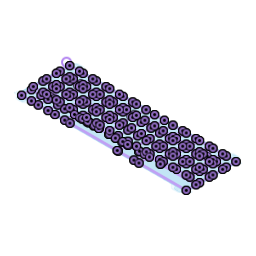
All_Plates (Autodesk Fusion 360 design; units mm, degrees)
Autodesk Fusion 360 part; units mm, degrees
(part 1 of 6)
sketch "campsite" plane through (0, 0, 0) normal (0, 1, 0) x (1, 0, 0)
  arc A0 (-6.7013, -67.15) -> (-8.4334, -66.15) centre (-8.4334, -68.15) ccw
  arc A1 (-9, 8.5) -> (-8.5, 9) centre (-8.5, 8.5) cw
  line L0 (-4.3919, 14) -> (3.6799, 14)
  arc A2 (-8.5, -66.15) -> (-9, -65.65) centre (-8.5, -65.65) cw
  line L1 (-8.5, 9) -> (-8.4334, 9)
  arc A3 (216.1161, 9) -> (217.8482, 10) centre (216.1161, 11) ccw
  line L2 (-6.7013, 10) -> (-4.3919, 14)
  line L3 (7.7214, 9) -> (216.1161, 9)
  arc A4 (-8.4334, 9) -> (-6.7013, 10) centre (-8.4334, 11) ccw
  arc A5 (232.8375, -65.65) -> (232.3375, -66.15) centre (232.3375, -65.65) cw
  line L4 (3.6799, 14) -> (5.9893, 10)
  line L5 (217.8482, 10) -> (220.1576, 14)
  line L6 (232.3375, -66.15) -> (232.2709, -66.15)
  line L7 (232.2709, 9) -> (232.3375, 9)
  arc A6 (217.8482, -67.15) -> (216.1161, -66.15) centre (216.1161, -68.15) ccw
  line L8 (-8.4334, -66.15) -> (-8.5, -66.15)
  arc A7 (7.7214, -66.15) -> (5.9893, -67.15) centre (7.7214, -68.15) ccw
  line L9 (220.1576, -71.15) -> (217.8482, -67.15)
  line L10 (-4.3919, -71.15) -> (-6.7013, -67.15)
  line L11 (-9, -65.65) -> (-9, 8.5)
  arc A8 (5.9893, 10) -> (7.7214, 9) centre (7.7214, 11) ccw
  arc A9 (232.2709, -66.15) -> (230.5388, -67.15) centre (232.2709, -68.15) ccw
  line L12 (232.8375, 8.5) -> (232.8375, -65.65)
  line L13 (228.2294, 14) -> (230.5388, 10)
  arc A10 (232.3375, 9) -> (232.8375, 8.5) centre (232.3375, 8.5) cw
  line L14 (5.9893, -67.15) -> (3.6799, -71.15)
  line L15 (216.1161, -66.15) -> (7.7214, -66.15)
  line L16 (228.2294, -71.15) -> (220.1576, -71.15)
  arc A11 (230.5388, 10) -> (232.2709, 9) centre (232.2709, 11) ccw
  line L17 (230.5388, -67.15) -> (228.2294, -71.15)
  line L18 (3.6799, -71.15) -> (-4.3919, -71.15)
  line L19 (220.1576, 14) -> (228.2294, 14)
sketch "coriander" plane through (0, 0, 0) normal (0, 1, 0) x (1, 0, 0)
  arc A0 (13.2901, -66.675) -> (10.6915, -67.7514) centre (13.2901, -70.35) ccw
  arc A1 (213.146, -67.7514) -> (210.5474, -66.675) centre (210.5474, -70.35) ccw
  line L0 (-9.525, -65.8599) -> (-9.525, 8.7099)
  arc A2 (226.5474, 15.525) -> (228.4389, 14.7415) centre (226.5474, 12.85) cw
  line L1 (228.4389, 14.7415) -> (232.579, 10.6014)
  line L2 (233.3625, 8.7099) -> (233.3625, -65.8599)
  arc A3 (232.579, 10.6014) -> (233.3625, 8.7099) centre (230.6875, 8.7099) cw
  line L3 (217.2861, -71.8915) -> (213.146, -67.7514)
  line L4 (213.114, 10.5694) -> (217.2861, 14.7415)
  line L5 (6.5514, 14.7415) -> (10.6915, 10.6014)
  arc A4 (-8.7415, -67.7514) -> (-9.525, -65.8599) centre (-6.85, -65.8599) cw
  arc A5 (210.5474, 9.525) -> (213.1139, 10.5697) centre (210.5474, 13.2) ccw
  arc A6 (10.6915, 10.6014) -> (13.2901, 9.525) centre (13.2901, 13.2) ccw
  arc A7 (-2.7099, -72.675) -> (-4.6014, -71.8915) centre (-2.7099, -70) cw
  arc A8 (6.5514, -71.8915) -> (4.6599, -72.675) centre (4.6599, -70) cw
  arc A9 (217.2861, 14.7415) -> (219.1776, 15.525) centre (219.1776, 12.85) cw
  line L6 (219.1776, 15.525) -> (226.5474, 15.525)
  arc A10 (228.4389, -71.8915) -> (226.5474, -72.675) centre (226.5474, -70) cw
  line L7 (10.6915, -67.7514) -> (6.5514, -71.8915)
  circle A11 centre (0.9751, -69.925) radius 1.25
  line L8 (-8.7415, 10.6014) -> (-4.6014, 14.7415)
  line L9 (232.579, -67.7514) -> (228.4389, -71.8915)
  arc A12 (-4.6014, 14.7415) -> (-2.7099, 15.525) centre (-2.7099, 12.85) cw
  arc A13 (233.3625, -65.8599) -> (232.579, -67.7514) centre (230.6875, -65.8599) cw
  arc A14 (219.1776, -72.675) -> (217.2861, -71.8915) centre (219.1776, -70) cw
  circle A15 centre (222.8626, -69.925) radius 1.25
  line L10 (-4.6014, -71.8915) -> (-8.7415, -67.7514)
  arc A16 (-9.525, 8.7099) -> (-8.7415, 10.6014) centre (-6.85, 8.7099) cw
  line L11 (-2.7099, 15.525) -> (4.6599, 15.525)
  line L12 (4.6599, -72.675) -> (-2.7099, -72.675)
  line L13 (226.5474, -72.675) -> (219.1776, -72.675)
  circle A17 centre (0.9749, 12.775) radius 1.25
  arc A18 (4.6599, 15.525) -> (6.5514, 14.7415) centre (4.6599, 12.85) cw
  line L14 (13.2901, 9.525) -> (210.5474, 9.525)
  arc A19 (213.1139, 10.5697) -> (213.114, 10.5694) centre (210.5375, 9.85) cw
  line L15 (210.5474, -66.675) -> (13.2901, -66.675)
  circle A20 centre (222.8624, 12.775) radius 1.25
sketch "hull" plane through (130.0399, 0, -35.1845) normal (0, 1, 0) x (1, 0, 0)
  arc A0 (107.0801, -27.1082) -> (107.0801, -29.5607) centre (107.3226, -28.3345) ccw
  arc A1 (104.8226, -31.0095) -> (103.3226, -32.5095) centre (104.8226, -32.5095) ccw
  line L0 (103.3226, -95.0095) -> (103.3226, -32.5095)
  line L1 (104.8226, -31.0095) -> (105.6476, -31.0095)
  arc A2 (105.6476, -31.0095) -> (107.2901, -30.4459) centre (105.6476, -28.3345) ccw
  arc A3 (107.2901, -30.4459) -> (107.0801, -29.5607) centre (106.9831, -30.0512) ccw
  arc A4 (-141.8899, -25.6595) -> (-143.5323, -26.2231) centre (-141.8899, -28.3345) ccw
  arc A5 (-143.3224, -29.5607) -> (-143.3224, -27.1082) centre (-143.5649, -28.3345) ccw
  arc A6 (-143.5323, -30.4459) -> (-141.8899, -31.0095) centre (-141.8899, -28.3345) ccw
  arc A7 (107.2901, -26.2231) -> (105.6476, -25.6595) centre (105.6476, -28.3345) ccw
  arc A8 (-139.5649, -32.5095) -> (-141.0649, -31.0095) centre (-141.0649, -32.5095) ccw
  arc A9 (107.0801, -27.1082) -> (107.2901, -26.2231) centre (106.9831, -26.6177) ccw
  line L2 (-139.5649, -32.5095) -> (-139.5649, -95.0095)
  line L3 (-141.0649, -96.5095) -> (-141.8899, -96.5095)
  arc A10 (-143.5323, -26.2231) -> (-143.3224, -27.1082) centre (-143.2253, -26.6177) ccw
  arc A11 (-143.3224, -29.5607) -> (-143.5323, -30.4459) centre (-143.2253, -30.0512) ccw
  line L4 (105.6476, -25.6595) -> (-141.8899, -25.6595)
  arc A12 (-141.0649, -96.5095) -> (-139.5649, -95.0095) centre (-141.0649, -95.0095) ccw
  line L5 (-141.8899, -31.0095) -> (-141.0649, -31.0095)
  arc A13 (107.2901, -101.2959) -> (107.0801, -100.4107) centre (106.9831, -100.9012) ccw
  arc A14 (107.2901, -97.0731) -> (105.6476, -96.5095) centre (105.6476, -99.1845) ccw
  arc A15 (-143.3224, -100.4107) -> (-143.3224, -97.9582) centre (-143.5649, -99.1845) ccw
  arc A16 (-141.8899, -96.5095) -> (-143.5323, -97.0731) centre (-141.8899, -99.1845) ccw
  arc A17 (-143.5323, -97.0731) -> (-143.3224, -97.9582) centre (-143.2253, -97.4677) ccw
  line L6 (-141.8899, -101.8595) -> (105.6476, -101.8595)
  arc A18 (103.3226, -95.0095) -> (104.8226, -96.5095) centre (104.8226, -95.0095) ccw
  arc A19 (-143.3224, -100.4107) -> (-143.5323, -101.2959) centre (-143.2253, -100.9012) ccw
  arc A20 (105.6476, -101.8595) -> (107.2901, -101.2959) centre (105.6476, -99.1845) ccw
  arc A21 (107.0801, -97.9582) -> (107.2901, -97.0731) centre (106.9831, -97.4677) ccw
  line L7 (105.6476, -96.5095) -> (104.8226, -96.5095)
  arc A22 (107.0801, -97.9582) -> (107.0801, -100.4107) centre (107.3226, -99.1845) ccw
  arc A23 (-143.5323, -101.2959) -> (-141.8899, -101.8595) centre (-141.8899, -99.1845) ccw
  point P0 (-130.0399, -35.1845)
sketch "tray" plane through (-50, 0, 0) normal (0, 1, 0) x (1, 0, 0)
  line L0 (43.225, 9.5245) -> (280.6123, 9.5245)
  line L1 (280.6123, -66.6754) -> (43.225, -66.6754)
  line L2 (283.6123, 6.5245) -> (283.6123, -63.6754)
  arc A0 (280.6123, 9.5245) -> (283.6123, 6.5245) centre (280.6123, 6.5245) cw
  arc A1 (283.6123, -63.6754) -> (280.6123, -66.6754) centre (280.6123, -63.6754) cw
  arc A2 (43.225, -66.6754) -> (40.225, -63.6754) centre (43.225, -63.6754) cw
  circle A3 centre (70.325, -44.2754) radius 2.75
  line L3 (40.225, -63.6754) -> (40.225, 6.5245)
  circle A4 centre (117.225, -55.8254) radius 2.75
  arc A5 (40.225, 6.5245) -> (43.225, 9.5245) centre (43.225, 6.5245) cw
  circle A6 centre (222.8123, -56.0254) radius 2.75
  circle A7 centre (251.1123, -7.2255) radius 2.75
  circle A8 centre (71.875, -9.5255) radius 2.75
  circle A9 centre (148.075, -9.5255) radius 2.75
  circle A10 centre (178.5623, -28.6255) radius 2.75
  point P0 (50, 0)
extrude "Extrude1" add sketch "campsite" along normal blind 10 makes body 1
extrude "Extrude2" add sketch "coriander" along normal blind 10 separate body contours A0 A1 L0 A2 L1 L2 A3 L3 L4 L5 A4 A6 A7 A8 A9 L6 A10 L7 L8 L9 A12 A13 A14 L10 A16 L11 L12 L13 A18 L14 A19 L15 | A5 L14 A19 picked at (210.945, 8.7857) makes body 2
extrude "Extrude3" add sketch "hull" along normal blind 10 separate body makes body 3
extrude "Extrude4" add sketch "tray" along normal blind 10 separate body makes body 4
copy_body "CopyPasteBodies1" bodies 2 makes body 5
move_body "Move1" bodies 5 to x (1, 0, 0) y (0, 1, 0) z (0, 0, 1) at (0, 0, 0)
combine "Combine1" operation intersect target body 5 tool bodies 1 keep tools
copy_body "CopyPasteBodies3" bodies 3 makes body 6
move_body "Move3" bodies 6 to x (1, 0, 0) y (0, 1, 0) z (0, 0, 1) at (0, 0, 0)
extrude "Extrude5" cut sketch "tray" along normal blind 10 contours A3 | A4 | A6 | A7 | A8 | A9 | A10 bodies 6
sketch "campiander" plane through (0, 0, 0) normal (0, 1, 0) x (1, 0, 0)
  line L0 (217.8482, 10) -> (220.1576, 14)
  arc A0 (-6.7013, -67.15) -> (-8.4334, -66.15) centre (-8.4334, -68.15) ccw
  line L1 (222.6139, -71.15) -> (220.1576, -71.15)
  line L2 (220.1576, -71.15) -> (217.8482, -67.15)
  arc A1 (222.6136, 14) -> (223.1111, 14) centre (222.8624, 12.775) ccw
  arc A2 (-8.5, -66.15) -> (-9, -65.65) centre (-8.5, -65.65) cw
  arc A3 (230.5388, 10) -> (232.2709, 9) centre (232.2709, 11) ccw
  arc A4 (-8.4334, 9) -> (-6.7013, 10) centre (-8.4334, 11) ccw
  arc A5 (217.8482, -67.15) -> (216.1161, -66.15) centre (216.1161, -68.15) ccw
  line L3 (232.3375, -66.15) -> (232.2709, -66.15)
  line L4 (-4.3919, 14) -> (0.7261, 14)
  line L5 (-9, -65.65) -> (-9, 8.5)
  line L6 (5.9893, -67.15) -> (3.6799, -71.15)
  line L7 (-8.4334, -66.15) -> (-8.5, -66.15)
  line L8 (-8.5, 9) -> (-8.4334, 9)
  line L9 (7.7214, 9) -> (216.1161, 9)
  arc A6 (232.2709, -66.15) -> (230.5388, -67.15) centre (232.2709, -68.15) ccw
  arc A7 (0.7261, 14) -> (1.2236, 14) centre (0.9749, 12.775) ccw
  arc A8 (1.2239, -71.15) -> (0.7264, -71.15) centre (0.9751, -69.925) ccw
  line L10 (223.1111, 14) -> (228.2294, 14)
  line L11 (228.2294, 14) -> (230.5388, 10)
  arc A9 (232.3375, 9) -> (232.8375, 8.5) centre (232.3375, 8.5) cw
  line L12 (232.8375, 8.5) -> (232.8375, -65.65)
  arc A10 (-9, 8.5) -> (-8.5, 9) centre (-8.5, 8.5) cw
  line L13 (-6.7013, 10) -> (-4.3919, 14)
  line L14 (0.7264, -71.15) -> (-4.3919, -71.15)
  line L15 (232.2709, 9) -> (232.3375, 9)
  line L16 (1.2236, 14) -> (3.6799, 14)
  line L17 (3.6799, 14) -> (5.9893, 10)
  arc A11 (216.1161, 9) -> (217.8482, 10) centre (216.1161, 11) ccw
  line L18 (220.1576, 14) -> (222.6136, 14)
  line L19 (228.2294, -71.15) -> (223.1114, -71.15)
  line L20 (230.5388, -67.15) -> (228.2294, -71.15)
  line L21 (3.6799, -71.15) -> (1.2239, -71.15)
  line L22 (216.1161, -66.15) -> (7.7214, -66.15)
  arc A12 (5.9893, 10) -> (7.7214, 9) centre (7.7214, 11) ccw
  arc A13 (232.8375, -65.65) -> (232.3375, -66.15) centre (232.3375, -65.65) cw
  arc A14 (7.7214, -66.15) -> (5.9893, -67.15) centre (7.7214, -68.15) ccw
  arc A15 (223.1114, -71.15) -> (222.6139, -71.15) centre (222.8626, -69.925) ccw
  line L23 (-4.3919, -71.15) -> (-6.7013, -67.15)
sketch "minisub" plane through (22.36, 0, 75.2938) normal (0, 1, 0) x (1, 0, 0)
  line L0 (52.5458, 11.1438) -> (52.5458, 26.1438)
  line L1 (115.6088, 25.1438) -> (101.6088, 25.1438)
  line L2 (208.4775, 11.1438) -> (208.4775, 25.1438)
  line L3 (140.8213, 26.1438) -> (140.8213, 25.1438)
  line L4 (45.5458, 26.1438) -> (40.8213, 26.1438)
  line L5 (76.4218, 26.1438) -> (69.4218, 26.1438)
  line L6 (100.1708, 26.1438) -> (93.1708, 26.1438)
  line L7 (52.5458, 26.1438) -> (47.8213, 26.1438)
  line L8 (100.1708, 11.1438) -> (101.6088, 11.1438)
  line L9 (147.8213, 26.1438) -> (140.8213, 26.1438)
  line L10 (147.8213, 25.1438) -> (147.8213, 26.1438)
  line L11 (67.9838, 25.1438) -> (53.9838, 25.1438)
  line L12 (148.9463, 11.1438) -> (148.9463, 25.1438)
  line L13 (47.8213, 11.1438) -> (52.5458, 11.1438)
  line L14 (101.6088, 25.1438) -> (100.1708, 25.1438)
  line L15 (208.4775, 25.1438) -> (194.4775, 25.1438)
  line L16 (47.8213, 26.1438) -> (45.5458, 26.1438)
  line L17 (53.9838, 11.1438) -> (67.9838, 11.1438)
  line L18 (115.6088, 11.1438) -> (115.6088, 25.1438)
  line L19 (147.8213, 11.1438) -> (148.9463, 11.1438)
  line L20 (124.0468, 11.1438) -> (124.0468, 26.1438)
  line L21 (175.4275, 11.1438) -> (189.4275, 11.1438)
  line L22 (69.4218, 11.1438) -> (76.4218, 11.1438)
  line L23 (194.4775, 25.1438) -> (194.4775, 11.1438)
  line L24 (189.4275, 11.1438) -> (189.4275, 25.1438)
  line L25 (93.1708, 25.1438) -> (87.3213, 25.1438)
  line L26 (189.4275, 25.1438) -> (175.4275, 25.1438)
  line L27 (69.4218, 26.1438) -> (69.4218, 11.1438)
  line L28 (170.3775, 25.1438) -> (156.3775, 25.1438)
  line L29 (93.1708, 26.1438) -> (93.1708, 25.1438)
  line L30 (156.3775, 11.1438) -> (170.3775, 11.1438)
  line L31 (93.1708, 11.1438) -> (100.1708, 11.1438)
  line L32 (53.9838, 25.1438) -> (53.9838, 11.1438)
  line L33 (45.5458, 11.1438) -> (47.8213, 11.1438)
  line L34 (124.0468, 26.1438) -> (117.0468, 26.1438)
  line L35 (140.8213, 25.1438) -> (134.9463, 25.1438)
  line L36 (175.4275, 25.1438) -> (175.4275, 11.1438)
  line L37 (117.0468, 11.1438) -> (124.0468, 11.1438)
  line L38 (76.4218, 11.1438) -> (76.4218, 26.1438)
  line L39 (140.8213, 11.1438) -> (147.8213, 11.1438)
  line L40 (134.9463, 11.1438) -> (140.8213, 11.1438)
  line L41 (65.89, 82.2938) -> (65.89, 68.2938)
  line L42 (142.09, 82.2938) -> (142.09, 68.2938)
  line L43 (175.14, 82.2938) -> (161.14, 82.2938)
  line L44 (46.84, 68.2938) -> (60.84, 68.2938)
  line L45 (84.94, 68.2938) -> (98.94, 68.2938)
  line L46 (8.74, 82.2938) -> (8.74, 68.2938)
  line L47 (117.99, 82.2938) -> (103.99, 82.2938)
  line L48 (98.94, 68.2938) -> (98.94, 82.2938)
  line L49 (123.04, 82.2938) -> (123.04, 68.2938)
  line L50 (41.79, 82.2938) -> (27.79, 82.2938)
  line L51 (79.89, 68.2938) -> (79.89, 82.2938)
  line L52 (27.79, 68.2938) -> (41.79, 68.2938)
  line L53 (161.14, 68.2938) -> (175.14, 68.2938)
  line L54 (13.5025, 49.2438) -> (27.5025, 49.2438)
  line L55 (175.14, 68.2938) -> (175.14, 82.2938)
  line L56 (46.84, 82.2938) -> (46.84, 68.2938)
  line L57 (65.89, 68.2938) -> (79.89, 68.2938)
  line L58 (103.99, 68.2938) -> (117.99, 68.2938)
  line L59 (41.79, 68.2938) -> (41.79, 82.2938)
  line L60 (98.94, 82.2938) -> (84.94, 82.2938)
  line L61 (117.99, 68.2938) -> (117.99, 82.2938)
  line L62 (142.09, 68.2938) -> (156.09, 68.2938)
  line L63 (60.84, 68.2938) -> (60.84, 82.2938)
  line L64 (22.74, 82.2938) -> (8.74, 82.2938)
  line L65 (156.09, 68.2938) -> (156.09, 82.2938)
  line L66 (187.3338, 68.2938) -> (201.3338, 68.2938)
  line L67 (3.69, 82.2938) -> (-10.31, 82.2938)
  line L68 (187.3338, 82.2938) -> (187.3338, 68.2938)
  line L69 (84.94, 82.2938) -> (84.94, 68.2938)
  line L70 (137.04, 82.2938) -> (123.04, 82.2938)
  line L71 (22.74, 68.2938) -> (22.74, 82.2938)
  line L72 (137.04, 68.2938) -> (137.04, 82.2938)
  line L73 (103.99, 82.2938) -> (103.99, 68.2938)
  line L74 (-10.31, 82.2938) -> (-10.31, 68.2938)
  line L75 (60.84, 82.2938) -> (46.84, 82.2938)
  line L76 (-26.9787, 49.2438) -> (-12.9787, 49.2438)
  line L77 (8.74, 68.2938) -> (22.74, 68.2938)
  line L78 (201.3338, 82.2938) -> (187.3338, 82.2938)
  line L79 (123.04, 68.2938) -> (137.04, 68.2938)
  line L80 (156.09, 82.2938) -> (142.09, 82.2938)
  line L81 (201.3338, 68.2938) -> (201.3338, 82.2938)
  line L82 (-12.9787, 63.2438) -> (-26.9787, 63.2438)
  line L83 (-12.9787, 49.2438) -> (-12.9787, 63.2438)
  line L84 (79.89, 82.2938) -> (65.89, 82.2938)
  line L85 (161.14, 82.2938) -> (161.14, 68.2938)
  line L86 (3.69, 68.2938) -> (3.69, 82.2938)
  line L87 (-26.9787, 63.2438) -> (-26.9787, 49.2438)
  line L88 (27.79, 82.2938) -> (27.79, 68.2938)
  line L89 (-5.5475, 49.2438) -> (8.4525, 49.2438)
  line L90 (8.4525, 49.2438) -> (8.4525, 63.2438)
  line L91 (-5.5475, 63.2438) -> (-5.5475, 49.2438)
  line L92 (8.4525, 63.2438) -> (-5.5475, 63.2438)
  line L93 (27.5025, 63.2438) -> (13.5025, 63.2438)
  line L94 (13.5025, 63.2438) -> (13.5025, 49.2438)
  line L95 (27.5025, 49.2438) -> (27.5025, 63.2438)
  line L96 (46.5525, 63.2438) -> (32.5525, 63.2438)
  line L97 (32.5525, 49.2438) -> (46.5525, 49.2438)
  line L98 (146.8525, 49.2438) -> (160.8525, 49.2438)
  line L99 (70.6525, 49.2438) -> (84.6525, 49.2438)
  line L100 (46.5525, 49.2438) -> (46.5525, 63.2438)
  line L101 (32.5525, 63.2438) -> (32.5525, 49.2438)
  line L102 (179.9025, 49.2438) -> (179.9025, 63.2438)
  line L103 (127.8025, 49.2438) -> (141.8025, 49.2438)
  line L104 (165.9025, 49.2438) -> (179.9025, 49.2438)
  line L105 (65.6025, 49.2438) -> (65.6025, 63.2438)
  line L106 (70.6525, 63.2438) -> (70.6525, 49.2438)
  line L107 (122.7525, 63.2438) -> (108.7525, 63.2438)
  line L108 (127.8025, 63.2438) -> (127.8025, 49.2438)
  line L109 (103.7025, 49.2438) -> (103.7025, 63.2438)
  line L110 (165.9025, 63.2438) -> (165.9025, 49.2438)
  line L111 (189.715, 49.2438) -> (203.715, 49.2438)
  line L112 (146.8525, 63.2438) -> (146.8525, 49.2438)
  line L113 (51.6025, 63.2438) -> (51.6025, 49.2438)
  line L114 (160.8525, 63.2438) -> (146.8525, 63.2438)
  line L115 (65.6025, 63.2438) -> (51.6025, 63.2438)
  line L116 (141.8025, 63.2438) -> (127.8025, 63.2438)
  line L117 (160.8525, 49.2438) -> (160.8525, 63.2438)
  line L118 (84.6525, 63.2438) -> (70.6525, 63.2438)
  line L119 (141.8025, 49.2438) -> (141.8025, 63.2438)
  line L120 (89.7025, 63.2438) -> (89.7025, 49.2438)
  line L121 (84.6525, 49.2438) -> (84.6525, 63.2438)
  line L122 (170.3775, 44.1938) -> (156.3775, 44.1938)
  line L123 (170.3775, 30.1938) -> (170.3775, 44.1938)
  line L124 (189.4275, 44.1938) -> (175.4275, 44.1938)
  line L125 (103.7025, 63.2438) -> (89.7025, 63.2438)
  line L126 (156.3775, 30.1938) -> (170.3775, 30.1938)
  line L127 (175.4275, 44.1938) -> (175.4275, 30.1938)
  line L128 (208.4775, 44.1938) -> (194.4775, 44.1938)
  line L129 (17.9775, 30.1938) -> (17.9775, 44.1938)
  line L130 (108.7525, 49.2438) -> (122.7525, 49.2438)
  line L131 (56.0775, 44.1938) -> (42.0775, 44.1938)
  line L132 (-8.2162, 30.1938) -> (-8.2162, 44.1938)
  line L133 (108.7525, 63.2438) -> (108.7525, 49.2438)
  line L134 (51.6025, 49.2438) -> (65.6025, 49.2438)
  line L135 (89.7025, 49.2438) -> (103.7025, 49.2438)
  line L136 (122.7525, 49.2438) -> (122.7525, 63.2438)
  line L137 (179.9025, 63.2438) -> (165.9025, 63.2438)
  line L138 (208.4775, 30.1938) -> (208.4775, 44.1938)
  line L139 (-12.9787, 11.1438) -> (-12.9787, 25.1438)
  line L140 (8.4525, 25.1438) -> (-5.5475, 25.1438)
  line L141 (80.1775, 30.1938) -> (94.1775, 30.1938)
  line L142 (99.2275, 44.1938) -> (99.2275, 30.1938)
  line L143 (175.4275, 30.1938) -> (189.4275, 30.1938)
  line L144 (8.4525, 11.1438) -> (8.4525, 25.1438)
  line L145 (-22.2162, 44.1938) -> (-22.2162, 30.1938)
  line L146 (137.3275, 44.1938) -> (137.3275, 30.1938)
  line L147 (-26.9787, 11.1438) -> (-12.9787, 11.1438)
  line L148 (-29.36, 68.2938) -> (-15.36, 68.2938)
  line L149 (-29.36, 82.2938) -> (-29.36, 68.2938)
  line L150 (-10.31, 68.2938) -> (3.69, 68.2938)
  line L151 (-15.36, 82.2938) -> (-29.36, 82.2938)
  line L152 (-15.36, 68.2938) -> (-15.36, 82.2938)
  line L153 (151.3275, 30.1938) -> (151.3275, 44.1938)
  line L154 (-8.2162, 44.1938) -> (-22.2162, 44.1938)
  line L155 (148.9463, 25.1438) -> (147.8213, 25.1438)
  line L156 (75.1275, 44.1938) -> (61.1275, 44.1938)
  line L157 (40.8213, 26.1438) -> (40.8213, 11.1438)
  line L158 (67.9838, 11.1438) -> (67.9838, 25.1438)
  line L159 (156.3775, 25.1438) -> (156.3775, 11.1438)
  line L160 (117.0468, 26.1438) -> (117.0468, 11.1438)
  line L161 (87.3213, 25.1438) -> (87.3213, 11.1438)
  line L162 (134.9463, 25.1438) -> (134.9463, 11.1438)
  line L163 (170.3775, 11.1438) -> (170.3775, 25.1438)
  line L164 (42.0775, 30.1938) -> (56.0775, 30.1938)
  line L165 (118.2775, 44.1938) -> (118.2775, 30.1938)
  line L166 (113.2275, 30.1938) -> (113.2275, 44.1938)
  line L167 (100.1708, 25.1438) -> (100.1708, 26.1438)
  line L168 (40.8213, 11.1438) -> (45.5458, 11.1438)
  line L169 (194.4775, 11.1438) -> (208.4775, 11.1438)
  line L170 (101.6088, 11.1438) -> (115.6088, 11.1438)
  line L171 (87.3213, 11.1438) -> (93.1708, 11.1438)
  line L172 (15.8838, 25.1438) -> (15.8838, 11.1438)
  line L173 (94.1775, 44.1938) -> (80.1775, 44.1938)
  line L174 (29.8838, 11.1438) -> (29.8838, 25.1438)
  line L175 (15.8838, 11.1438) -> (29.8838, 11.1438)
  line L176 (-5.5475, 25.1438) -> (-5.5475, 11.1438)
  line L177 (203.715, 63.2438) -> (189.715, 63.2438)
  line L178 (189.4275, 30.1938) -> (189.4275, 44.1938)
  line L179 (156.3775, 44.1938) -> (156.3775, 30.1938)
  line L180 (194.4775, 30.1938) -> (208.4775, 30.1938)
  line L181 (29.8838, 25.1438) -> (15.8838, 25.1438)
  line L182 (194.4775, 44.1938) -> (194.4775, 30.1938)
  line L183 (-5.5475, 11.1438) -> (8.4525, 11.1438)
  line L184 (-12.9787, 25.1438) -> (-26.9787, 25.1438)
  line L185 (3.9775, 44.1938) -> (3.9775, 30.1938)
  line L186 (-26.9787, 25.1438) -> (-26.9787, 11.1438)
  line L187 (37.0275, 30.1938) -> (37.0275, 44.1938)
  line L188 (3.9775, 30.1938) -> (17.9775, 30.1938)
  line L189 (23.0275, 30.1938) -> (37.0275, 30.1938)
  line L190 (61.1275, 44.1938) -> (61.1275, 30.1938)
  line L191 (42.0775, 44.1938) -> (42.0775, 30.1938)
  line L192 (94.1775, 30.1938) -> (94.1775, 44.1938)
  line L193 (189.715, 63.2438) -> (189.715, 49.2438)
  line L194 (17.9775, 44.1938) -> (3.9775, 44.1938)
  line L195 (99.2275, 30.1938) -> (113.2275, 30.1938)
  line L196 (132.2775, 44.1938) -> (118.2775, 44.1938)
  line L197 (132.2775, 30.1938) -> (132.2775, 44.1938)
  line L198 (-22.2162, 30.1938) -> (-8.2162, 30.1938)
  line L199 (75.1275, 30.1938) -> (75.1275, 44.1938)
  line L200 (61.1275, 30.1938) -> (75.1275, 30.1938)
  line L201 (80.1775, 44.1938) -> (80.1775, 30.1938)
  line L202 (203.715, 49.2438) -> (203.715, 63.2438)
  line L203 (37.0275, 44.1938) -> (23.0275, 44.1938)
  line L204 (137.3275, 30.1938) -> (151.3275, 30.1938)
  line L205 (23.0275, 44.1938) -> (23.0275, 30.1938)
  line L206 (56.0775, 30.1938) -> (56.0775, 44.1938)
  line L207 (151.3275, 44.1938) -> (137.3275, 44.1938)
  line L208 (113.2275, 44.1938) -> (99.2275, 44.1938)
  line L209 (118.2775, 30.1938) -> (132.2775, 30.1938)
  point P0 (-22.36, 75.2938)
sketch "jetvan" plane through (-13.4449, 0, -95.9528) normal (0, 1, 0) x (1, 0, 0)
  line L0 (20.4449, -88.9528) -> (6.4449, -88.9528)
  line L1 (6.4449, -102.9528) -> (20.4449, -102.9528)
  line L2 (115.6949, -88.9528) -> (101.6949, -88.9528)
  line L3 (120.7449, -102.9528) -> (134.7449, -102.9528)
  line L4 (77.5949, -102.9528) -> (77.5949, -88.9528)
  line L5 (82.6449, -102.9528) -> (96.6449, -102.9528)
  line L6 (158.8449, -102.9528) -> (172.8449, -102.9528)
  line L7 (20.4449, -102.9528) -> (20.4449, -88.9528)
  line L8 (63.5949, -88.9528) -> (63.5949, -102.9528)
  line L9 (82.6449, -88.9528) -> (82.6449, -102.9528)
  line L10 (44.5449, -102.9528) -> (58.5449, -102.9528)
  line L11 (115.6949, -102.9528) -> (115.6949, -88.9528)
  line L12 (6.4449, -88.9528) -> (6.4449, -102.9528)
  line L13 (101.6949, -88.9528) -> (101.6949, -102.9528)
  line L14 (177.8949, -88.9528) -> (177.8949, -102.9528)
  line L15 (101.6949, -102.9528) -> (115.6949, -102.9528)
  line L16 (153.7949, -102.9528) -> (153.7949, -88.9528)
  line L17 (191.8949, -102.9528) -> (191.8949, -88.9528)
  line L18 (58.5449, -88.9528) -> (44.5449, -88.9528)
  line L19 (134.7449, -88.9528) -> (120.7449, -88.9528)
  line L20 (153.7949, -88.9528) -> (139.7949, -88.9528)
  line L21 (177.8949, -102.9528) -> (191.8949, -102.9528)
  line L22 (191.8949, -88.9528) -> (177.8949, -88.9528)
  line L23 (172.8449, -102.9528) -> (172.8449, -88.9528)
  line L24 (158.8449, -88.9528) -> (158.8449, -102.9528)
  line L25 (134.7449, -102.9528) -> (134.7449, -88.9528)
  line L26 (63.5949, -102.9528) -> (77.5949, -102.9528)
  line L27 (120.7449, -88.9528) -> (120.7449, -102.9528)
  line L28 (39.4949, -102.9528) -> (39.4949, -88.9528)
  line L29 (196.9449, -102.9528) -> (210.9449, -102.9528)
  line L30 (172.8449, -88.9528) -> (158.8449, -88.9528)
  line L31 (210.9449, -88.9528) -> (196.9449, -88.9528)
  line L32 (139.7949, -88.9528) -> (139.7949, -102.9528)
  line L33 (139.7949, -102.9528) -> (153.7949, -102.9528)
  line L34 (39.4949, -88.9528) -> (25.4949, -88.9528)
  line L35 (77.5949, -88.9528) -> (63.5949, -88.9528)
  line L36 (44.5449, -88.9528) -> (44.5449, -102.9528)
  line L37 (30.2574, -108.0028) -> (30.2574, -122.0028)
  line L38 (158.5574, -122.0028) -> (158.5574, -108.0028)
  line L39 (129.9824, -141.0528) -> (129.9824, -127.0528)
  line L40 (68.3574, -122.0028) -> (82.3574, -122.0028)
  line L41 (225.5199, -122.0028) -> (239.5199, -122.0028)
  line L42 (22.8262, -108.0028) -> (8.8262, -108.0028)
  line L43 (101.4074, -122.0028) -> (101.4074, -108.0028)
  line L44 (139.5074, -108.0028) -> (125.5074, -108.0028)
  line L45 (25.4949, -88.9528) -> (25.4949, -102.9528)
  line L46 (196.9449, -88.9528) -> (196.9449, -102.9528)
  line L47 (223.1387, -102.9528) -> (237.1387, -102.9528)
  line L48 (237.1387, -102.9528) -> (237.1387, -88.9528)
  line L49 (22.8262, -122.0028) -> (22.8262, -108.0028)
  line L50 (44.2574, -108.0028) -> (30.2574, -108.0028)
  line L51 (63.3074, -108.0028) -> (49.3074, -108.0028)
  line L52 (68.3574, -108.0028) -> (68.3574, -122.0028)
  line L53 (96.6449, -102.9528) -> (96.6449, -88.9528)
  line L54 (101.4074, -108.0028) -> (87.4074, -108.0028)
  line L55 (53.7824, -127.0528) -> (39.7824, -127.0528)
  line L56 (192.1824, -141.0528) -> (206.1824, -141.0528)
  line L57 (206.1824, -127.0528) -> (192.1824, -127.0528)
  line L58 (120.4574, -108.0028) -> (106.4574, -108.0028)
  line L59 (30.2574, -122.0028) -> (44.2574, -122.0028)
  line L60 (192.1824, -127.0528) -> (192.1824, -141.0528)
  line L61 (44.2574, -122.0028) -> (44.2574, -108.0028)
  line L62 (27.5887, -127.0528) -> (13.5887, -127.0528)
  line L63 (82.3574, -122.0028) -> (82.3574, -108.0028)
  line L64 (25.4949, -102.9528) -> (39.4949, -102.9528)
  line L65 (8.8262, -122.0028) -> (22.8262, -122.0028)
  line L66 (49.3074, -122.0028) -> (63.3074, -122.0028)
  line L67 (82.3574, -108.0028) -> (68.3574, -108.0028)
  line L68 (144.5574, -122.0028) -> (158.5574, -122.0028)
  line L69 (87.4074, -108.0028) -> (87.4074, -122.0028)
  line L70 (106.4574, -108.0028) -> (106.4574, -122.0028)
  line L71 (187.1324, -141.0528) -> (187.1324, -127.0528)
  line L72 (182.6574, -122.0028) -> (196.6574, -122.0028)
  line L73 (139.5074, -122.0028) -> (139.5074, -108.0028)
  line L74 (182.6574, -108.0028) -> (182.6574, -122.0028)
  line L75 (223.1387, -88.9528) -> (223.1387, -102.9528)
  line L76 (196.6574, -122.0028) -> (196.6574, -108.0028)
  line L77 (239.5199, -122.0028) -> (239.5199, -108.0028)
  line L78 (125.5074, -122.0028) -> (139.5074, -122.0028)
  line L79 (237.1387, -88.9528) -> (223.1387, -88.9528)
  line L80 (158.5574, -108.0028) -> (144.5574, -108.0028)
  line L81 (49.3074, -108.0028) -> (49.3074, -122.0028)
  line L82 (87.4074, -122.0028) -> (101.4074, -122.0028)
  line L83 (106.4574, -122.0028) -> (120.4574, -122.0028)
  line L84 (173.1324, -127.0528) -> (173.1324, -141.0528)
  line L85 (77.8824, -141.0528) -> (91.8824, -141.0528)
  line L86 (168.0824, -127.0528) -> (154.0824, -127.0528)
  line L87 (210.9449, -102.9528) -> (210.9449, -88.9528)
  line L88 (96.6449, -88.9528) -> (82.6449, -88.9528)
  line L89 (63.3074, -122.0028) -> (63.3074, -108.0028)
  line L90 (125.5074, -108.0028) -> (125.5074, -122.0028)
  line L91 (163.6074, -122.0028) -> (177.6074, -122.0028)
  line L92 (8.8262, -108.0028) -> (8.8262, -122.0028)
  line L93 (120.4574, -122.0028) -> (120.4574, -108.0028)
  line L94 (144.5574, -108.0028) -> (144.5574, -122.0028)
  line L95 (91.8824, -141.0528) -> (91.8824, -127.0528)
  line L96 (58.5449, -102.9528) -> (58.5449, -88.9528)
  line L97 (39.7824, -141.0528) -> (53.7824, -141.0528)
  line L98 (225.2324, -141.0528) -> (225.2324, -127.0528)
  line L99 (110.9324, -127.0528) -> (96.9324, -127.0528)
  line L100 (91.8824, -127.0528) -> (77.8824, -127.0528)
  line L101 (201.7074, -122.0028) -> (215.7074, -122.0028)
  line L102 (168.0824, -141.0528) -> (168.0824, -127.0528)
  line L103 (154.0824, -141.0528) -> (168.0824, -141.0528)
  line L104 (154.0824, -127.0528) -> (154.0824, -141.0528)
  line L105 (230.2824, -160.1028) -> (244.2824, -160.1028)
  line L106 (201.7074, -108.0028) -> (201.7074, -122.0028)
  line L107 (72.8324, -127.0528) -> (58.8324, -127.0528)
  line L108 (76.6262, -160.1028) -> (83.6262, -160.1028)
  line L109 (13.5887, -141.0528) -> (27.5887, -141.0528)
  line L110 (177.6074, -108.0028) -> (163.6074, -108.0028)
  line L111 (244.2824, -141.0528) -> (244.2824, -127.0528)
  line L112 (135.0324, -141.0528) -> (149.0324, -141.0528)
  line L113 (239.5199, -108.0028) -> (225.5199, -108.0028)
  line L114 (22.8262, -160.1028) -> (22.8262, -146.1028)
  line L115 (225.2324, -127.0528) -> (211.2324, -127.0528)
  line L116 (225.5199, -108.0028) -> (225.5199, -122.0028)
  line L117 (123.1262, -146.1028) -> (123.1262, -160.1028)
  line L118 (51.6887, -146.1028) -> (51.6887, -160.1028)
  line L119 (137.1262, -146.1028) -> (123.1262, -146.1028)
  line L120 (187.1324, -127.0528) -> (173.1324, -127.0528)
  line L121 (27.5887, -141.0528) -> (27.5887, -127.0528)
  line L122 (96.9324, -141.0528) -> (110.9324, -141.0528)
  line L123 (192.1824, -160.1028) -> (206.1824, -160.1028)
  line L124 (177.6074, -122.0028) -> (177.6074, -108.0028)
  line L125 (211.2324, -141.0528) -> (225.2324, -141.0528)
  line L126 (83.6262, -145.1028) -> (76.6262, -145.1028)
  line L127 (211.2324, -160.1028) -> (225.2324, -160.1028)
  line L128 (230.2824, -146.1028) -> (230.2824, -160.1028)
  line L129 (129.9824, -127.0528) -> (115.9824, -127.0528)
  line L130 (96.9324, -127.0528) -> (96.9324, -141.0528)
  line L131 (244.2824, -127.0528) -> (230.2824, -127.0528)
  line L132 (163.6074, -108.0028) -> (163.6074, -122.0028)
  line L133 (196.6574, -108.0028) -> (182.6574, -108.0028)
  line L134 (149.0324, -141.0528) -> (149.0324, -127.0528)
  line L135 (230.2824, -141.0528) -> (244.2824, -141.0528)
  line L136 (39.7824, -127.0528) -> (39.7824, -141.0528)
  line L137 (115.9824, -141.0528) -> (129.9824, -141.0528)
  line L138 (77.8824, -127.0528) -> (77.8824, -141.0528)
  line L139 (176.6262, -160.1028) -> (183.6262, -160.1028)
  line L140 (215.7074, -108.0028) -> (201.7074, -108.0028)
  line L141 (211.2324, -146.1028) -> (211.2324, -160.1028)
  line L142 (58.8324, -127.0528) -> (58.8324, -141.0528)
  line L143 (72.8324, -141.0528) -> (72.8324, -127.0528)
  line L144 (211.2324, -127.0528) -> (211.2324, -141.0528)
  line L145 (110.9324, -141.0528) -> (110.9324, -127.0528)
  line L146 (115.9824, -127.0528) -> (115.9824, -141.0528)
  line L147 (149.0324, -127.0528) -> (135.0324, -127.0528)
  line L148 (58.8324, -141.0528) -> (72.8324, -141.0528)
  line L149 (8.8262, -160.1028) -> (22.8262, -160.1028)
  line L150 (230.2824, -127.0528) -> (230.2824, -141.0528)
  line L151 (206.1824, -141.0528) -> (206.1824, -127.0528)
  line L152 (135.0324, -127.0528) -> (135.0324, -141.0528)
  line L153 (53.7824, -141.0528) -> (53.7824, -127.0528)
  line L154 (51.6887, -160.1028) -> (65.6887, -160.1028)
  line L155 (137.1262, -160.1028) -> (137.1262, -146.1028)
  line L156 (173.1324, -141.0528) -> (187.1324, -141.0528)
  line L157 (192.1824, -146.1028) -> (192.1824, -160.1028)
  line L158 (30.2574, -146.1028) -> (30.2574, -160.1028)
  line L159 (13.5887, -127.0528) -> (13.5887, -141.0528)
  line L160 (215.7074, -122.0028) -> (215.7074, -108.0028)
  line L161 (206.1824, -146.1028) -> (192.1824, -146.1028)
  line L162 (123.1262, -160.1028) -> (137.1262, -160.1028)
  line L163 (176.6262, -145.1028) -> (176.6262, -160.1028)
  line L164 (225.2324, -146.1028) -> (211.2324, -146.1028)
  line L165 (22.8262, -146.1028) -> (8.8262, -146.1028)
  line L166 (83.6262, -160.1028) -> (83.6262, -145.1028)
  line L167 (244.2824, -160.1028) -> (244.2824, -146.1028)
  line L168 (44.2574, -146.1028) -> (30.2574, -146.1028)
  line L169 (65.6887, -160.1028) -> (65.6887, -146.1028)
  line L170 (30.2574, -160.1028) -> (44.2574, -160.1028)
  line L171 (225.2324, -160.1028) -> (225.2324, -146.1028)
  line L172 (183.6262, -160.1028) -> (183.6262, -145.1028)
  line L173 (76.6262, -145.1028) -> (76.6262, -160.1028)
  line L174 (65.6887, -146.1028) -> (51.6887, -146.1028)
  line L175 (8.8262, -146.1028) -> (8.8262, -160.1028)
  line L176 (206.1824, -160.1028) -> (206.1824, -146.1028)
  line L177 (44.2574, -160.1028) -> (44.2574, -146.1028)
  line L178 (183.6262, -145.1028) -> (176.6262, -145.1028)
  line L179 (244.2824, -146.1028) -> (230.2824, -146.1028)
  point P0 (13.4449, -95.9528)
sketch "ketch" plane through (0, 0, 0) normal (0, 1, 0) x (1, 0, 0)
  line L0 (109.6813, -50.15) -> (109.6813, -64.15)
  line L1 (123.6813, -50.15) -> (121.5875, -50.15)
  line L2 (120.1495, -64.15) -> (121.5875, -64.15)
  line L3 (113.1495, -64.15) -> (120.1495, -64.15)
  line L4 (121.5875, -50.15) -> (120.1495, -50.15)
  line L5 (113.1495, -50.15) -> (109.6813, -50.15)
  line L6 (26.05, -7) -> (26.05, 7)
  line L7 (31.1, 7) -> (31.1, -7)
  line L8 (64.15, 7) -> (50.15, 7)
  line L9 (50.15, 7) -> (50.15, -7)
  line L10 (64.15, -7) -> (64.15, 7)
  line L11 (83.2, -7) -> (83.2, 7)
  line L12 (88.25, -7) -> (102.25, -7)
  line L13 (7, -7) -> (7, 7)
  line L14 (-7, -7) -> (7, -7)
  line L15 (45.1, 7) -> (31.1, 7)
  line L16 (69.2, 7) -> (69.2, -7)
  line L17 (50.15, -7) -> (64.15, -7)
  line L18 (26.05, 7) -> (12.05, 7)
  line L19 (7, 7) -> (-7, 7)
  line L20 (45.1, -7) -> (45.1, 7)
  line L21 (12.05, 7) -> (12.05, -7)
  line L22 (69.2, -7) -> (83.2, -7)
  line L23 (83.2, 7) -> (69.2, 7)
  line L24 (-7, 7) -> (-7, -7)
  line L25 (12.05, -7) -> (26.05, -7)
  line L26 (102.25, 7) -> (88.25, 7)
  line L27 (31.1, -7) -> (45.1, -7)
  line L28 (102.25, -7) -> (102.25, 7)
  line L29 (164.1625, -12.05) -> (150.1625, -12.05)
  line L30 (145.1125, -12.05) -> (131.1125, -12.05)
  line L31 (140.35, 7) -> (126.35, 7)
  line L32 (188.2625, -12.05) -> (188.2625, -26.05)
  line L33 (212.075, -12.05) -> (212.075, -26.05)
  line L34 (164.1625, -26.05) -> (164.1625, -12.05)
  line L35 (121.3, 7) -> (107.3, 7)
  line L36 (159.4, -7) -> (159.4, 7)
  line L37 (-4.6187, -12.05) -> (-4.6187, -26.05)
  line L38 (131.1125, -12.05) -> (131.1125, -26.05)
  line L39 (145.4, 7) -> (145.4, -7)
  line L40 (164.45, 7) -> (164.45, -7)
  line L41 (107.3, -7) -> (121.3, -7)
  line L42 (9.3813, -26.05) -> (9.3813, -12.05)
  line L43 (35.8625, -12.05) -> (35.8625, -26.05)
  line L44 (150.1625, -12.05) -> (150.1625, -26.05)
  line L45 (-4.6187, -26.05) -> (9.3813, -26.05)
  line L46 (183.2125, -12.05) -> (169.2125, -12.05)
  line L47 (226.075, -12.05) -> (212.075, -12.05)
  line L48 (202.2625, -26.05) -> (202.2625, -12.05)
  line L49 (140.35, -7) -> (140.35, 7)
  line L50 (197.5, 7) -> (183.5, 7)
  line L51 (68.9125, -12.05) -> (54.9125, -12.05)
  line L52 (68.9125, -26.05) -> (68.9125, -12.05)
  line L53 (121.3, -7) -> (121.3, 7)
  line L54 (178.45, -7) -> (178.45, 7)
  line L55 (145.1125, -26.05) -> (145.1125, -12.05)
  line L56 (164.45, -7) -> (178.45, -7)
  line L57 (145.4, -7) -> (159.4, -7)
  line L58 (183.5, 7) -> (183.5, -7)
  line L59 (49.8625, -12.05) -> (35.8625, -12.05)
  line L60 (49.8625, -26.05) -> (49.8625, -12.05)
  line L61 (226.075, -26.05) -> (226.075, -12.05)
  line L62 (131.1125, -26.05) -> (145.1125, -26.05)
  line L63 (188.2625, -26.05) -> (202.2625, -26.05)
  line L64 (126.35, 7) -> (126.35, -7)
  line L65 (197.5, -7) -> (197.5, 7)
  line L66 (223.6938, 7) -> (209.6937, 7)
  line L67 (209.6937, 7) -> (209.6937, -7)
  line L68 (183.5, -7) -> (197.5, -7)
  line L69 (107.0125, -26.05) -> (107.0125, -12.05)
  line L70 (107.3, 7) -> (107.3, -7)
  line L71 (126.35, -7) -> (140.35, -7)
  line L72 (223.6938, -7) -> (223.6938, 7)
  line L73 (88.25, 7) -> (88.25, -7)
  line L74 (178.45, 7) -> (164.45, 7)
  line L75 (30.8125, -12.05) -> (16.8125, -12.05)
  line L76 (30.8125, -26.05) -> (30.8125, -12.05)
  line L77 (16.8125, -12.05) -> (16.8125, -26.05)
  line L78 (35.8625, -26.05) -> (49.8625, -26.05)
  line L79 (54.9125, -26.05) -> (68.9125, -26.05)
  line L80 (209.6937, -7) -> (223.6938, -7)
  line L81 (159.4, 7) -> (145.4, 7)
  line L82 (16.8125, -26.05) -> (30.8125, -26.05)
  line L83 (9.3813, -12.05) -> (-4.6187, -12.05)
  line L84 (54.9125, -12.05) -> (54.9125, -26.05)
  line L85 (107.0125, -12.05) -> (93.0125, -12.05)
  line L86 (78.4375, -31.1) -> (64.4375, -31.1)
  line L87 (112.0625, -12.05) -> (112.0625, -26.05)
  line L88 (12.05, -64.15) -> (16.8125, -64.15)
  line L89 (59.3875, -45.1) -> (59.3875, -31.1)
  line L90 (64.4375, -45.1) -> (78.4375, -45.1)
  line L91 (83.4875, -45.1) -> (97.4875, -45.1)
  line L92 (0.1438, -45.1) -> (14.1438, -45.1)
  line L93 (26.3375, -31.1) -> (26.3375, -45.1)
  line L94 (16.8125, -50.15) -> (12.05, -50.15)
  line L95 (150.1625, -26.05) -> (164.1625, -26.05)
  line L96 (59.3875, -31.1) -> (45.3875, -31.1)
  line L97 (169.2125, -26.05) -> (183.2125, -26.05)
  line L98 (183.2125, -26.05) -> (183.2125, -12.05)
  line L99 (45.1, -50.15) -> (38.2437, -50.15)
  line L100 (30.8125, -64.15) -> (31.1, -64.15)
  line L101 (14.1437, -45.1) -> (14.1437, -31.1)
  line L102 (159.6875, -31.1) -> (159.6875, -45.1)
  line L103 (87.9625, -12.05) -> (73.9625, -12.05)
  line L104 (14.1437, -31.1) -> (0.1437, -31.1)
  line L105 (93.0125, -26.05) -> (107.0125, -26.05)
  line L106 (0.1438, -31.1) -> (0.1438, -45.1)
  line L107 (73.9625, -12.05) -> (73.9625, -26.05)
  line L108 (45.3875, -45.1) -> (59.3875, -45.1)
  line L109 (64.4375, -31.1) -> (64.4375, -45.1)
  line L110 (40.3375, -31.1) -> (26.3375, -31.1)
  line L111 (212.075, -26.05) -> (226.075, -26.05)
  line L112 (112.0625, -26.05) -> (126.0625, -26.05)
  line L113 (126.0625, -12.05) -> (112.0625, -12.05)
  line L114 (140.6375, -31.1) -> (140.6375, -45.1)
  line L115 (45.3875, -31.1) -> (45.3875, -45.1)
  line L116 (169.2125, -12.05) -> (169.2125, -26.05)
  line L117 (73.9625, -26.05) -> (87.9625, -26.05)
  line L118 (126.0625, -26.05) -> (126.0625, -12.05)
  line L119 (9.3813, -64.15) -> (9.3813, -50.15)
  line L120 (93.0125, -12.05) -> (93.0125, -26.05)
  line L121 (197.7875, -45.1) -> (211.7875, -45.1)
  line L122 (202.2625, -12.05) -> (188.2625, -12.05)
  line L123 (87.9625, -26.05) -> (87.9625, -12.05)
  line L124 (26.3375, -45.1) -> (40.3375, -45.1)
  line L125 (78.4375, -45.1) -> (78.4375, -31.1)
  line L126 (40.3375, -45.1) -> (40.3375, -31.1)
  line L127 (-4.6187, -50.15) -> (-7, -50.15)
  line L128 (-7, -64.15) -> (-4.6187, -64.15)
  line L129 (116.5375, -45.1) -> (116.5375, -31.1)
  line L130 (31.1, -64.15) -> (35.575, -64.15)
  line L131 (97.4875, -45.1) -> (97.4875, -31.1)
  line L132 (47.7688, -64.15) -> (50.15, -64.15)
  line L133 (230.8375, -45.1) -> (230.8375, -31.1)
  line L134 (7, -50.15) -> (-4.6187, -50.15)
  line L135 (-7, -50.15) -> (-7, -64.15)
  line L136 (178.7375, -45.1) -> (192.7375, -45.1)
  line L137 (31.1, -50.15) -> (30.8125, -50.15)
  line L138 (16.8125, -64.15) -> (21.575, -64.15)
  line L139 (35.575, -64.15) -> (38.2437, -64.15)
  line L140 (197.7875, -31.1) -> (197.7875, -45.1)
  line L141 (35.575, -50.15) -> (31.1, -50.15)
  line L142 (38.2437, -50.15) -> (35.575, -50.15)
  line L143 (50.15, -64.15) -> (52.2438, -64.15)
  line L144 (216.8375, -31.1) -> (216.8375, -45.1)
  line L145 (211.7875, -31.1) -> (197.7875, -31.1)
  line L146 (116.5375, -31.1) -> (102.5375, -31.1)
  line L147 (211.7875, -45.1) -> (211.7875, -31.1)
  line L148 (173.6875, -45.1) -> (173.6875, -31.1)
  line L149 (192.7375, -45.1) -> (192.7375, -31.1)
  line L150 (30.8125, -50.15) -> (26.05, -50.15)
  line L151 (9.3813, -50.15) -> (7, -50.15)
  line L152 (121.5875, -31.1) -> (121.5875, -45.1)
  line L153 (50.15, -50.15) -> (47.7688, -50.15)
  line L154 (83.4875, -31.1) -> (83.4875, -45.1)
  line L155 (102.5375, -31.1) -> (102.5375, -45.1)
  line L156 (230.8375, -31.1) -> (216.8375, -31.1)
  line L157 (216.8375, -45.1) -> (230.8375, -45.1)
  line L158 (121.5875, -45.1) -> (135.5875, -45.1)
  line L159 (47.7688, -50.15) -> (45.1, -50.15)
  line L160 (7, -64.15) -> (9.3813, -64.15)
  line L161 (135.5875, -45.1) -> (135.5875, -31.1)
  line L162 (140.6375, -45.1) -> (154.6375, -45.1)
  line L163 (81.1062, -64.15) -> (95.1062, -64.15)
  line L164 (154.925, -64.15) -> (163.1813, -64.15)
  line L165 (26.05, -50.15) -> (21.575, -50.15)
  line L166 (154.6375, -45.1) -> (154.6375, -31.1)
  line L167 (173.6875, -31.1) -> (159.6875, -31.1)
  line L168 (216.8375, -64.15) -> (223.6938, -64.15)
  line L169 (103.5442, -64.15) -> (103.5442, -49.15)
  line L170 (63.1813, -49.15) -> (63.1813, -50.15)
  line L171 (70.1813, -49.15) -> (63.1813, -49.15)
  line L172 (72.6683, -49.15) -> (72.6683, -64.15)
  line L173 (63.1813, -64.15) -> (64.15, -64.15)
  line L174 (21.575, -64.15) -> (26.05, -64.15)
  line L175 (135.5875, -64.15) -> (135.5875, -50.15)
  line L176 (135.5875, -31.1) -> (121.5875, -31.1)
  line L177 (120.1495, -50.15) -> (120.1495, -49.15)
  line L178 (109.6813, -64.15) -> (113.1495, -64.15)
  line L179 (192.7375, -31.1) -> (178.7375, -31.1)
  line L180 (12.05, -50.15) -> (12.05, -64.15)
  line L181 (45.1, -64.15) -> (47.7688, -64.15)
  line L182 (52.2438, -64.15) -> (61.7688, -64.15)
  line L183 (121.5875, -64.15) -> (123.6813, -64.15)
  line L184 (21.575, -50.15) -> (16.8125, -50.15)
  line L185 (97.4875, -31.1) -> (83.4875, -31.1)
  line L186 (144.0255, -49.15) -> (137.0255, -49.15)
  line L187 (178.7375, -31.1) -> (178.7375, -45.1)
  line L188 (163.1813, -64.15) -> (166.5437, -64.15)
  line L189 (-4.6187, -64.15) -> (7, -64.15)
  line L190 (144.0255, -64.15) -> (144.0255, -49.15)
  line L191 (52.2438, -50.15) -> (50.15, -50.15)
  line L192 (102.5375, -45.1) -> (116.5375, -45.1)
  line L193 (79.6683, -64.15) -> (79.6683, -49.15)
  line L194 (137.0255, -64.15) -> (144.0255, -64.15)
  line L195 (96.5443, -49.15) -> (96.5443, -64.15)
  line L196 (154.6375, -31.1) -> (140.6375, -31.1)
  line L197 (61.7688, -64.15) -> (63.1813, -64.15)
  line L198 (38.2437, -64.15) -> (45.1, -64.15)
  line L199 (61.7688, -50.15) -> (52.2438, -50.15)
  line L200 (166.5437, -64.15) -> (168.925, -64.15)
  line L201 (26.05, -64.15) -> (30.8125, -64.15)
  line L202 (168.925, -64.15) -> (170.1813, -64.15)
  line L203 (63.1813, -50.15) -> (61.7688, -50.15)
  line L204 (113.1495, -49.15) -> (113.1495, -50.15)
  line L205 (64.15, -64.15) -> (70.1813, -64.15)
  line L206 (137.0255, -49.15) -> (137.0255, -64.15)
  line L207 (79.6683, -49.15) -> (72.6683, -49.15)
  line L208 (120.1495, -49.15) -> (113.1495, -49.15)
  line L209 (152.5437, -64.15) -> (154.925, -64.15)
  line L210 (159.6875, -45.1) -> (173.6875, -45.1)
  line L211 (163.1813, -50.15) -> (154.925, -50.15)
  line L212 (192.7375, -50.15) -> (178.7375, -50.15)
  line L213 (81.1062, -50.15) -> (81.1062, -64.15)
  line L214 (163.1813, -49.15) -> (163.1813, -50.15)
  line L215 (223.6938, -64.15) -> (230.8375, -64.15)
  line L216 (70.1813, -64.15) -> (70.1813, -49.15)
  line L217 (197.7875, -64.15) -> (209.6937, -64.15)
  line L218 (178.7375, -64.15) -> (192.7375, -64.15)
  line L219 (72.6683, -64.15) -> (79.6683, -64.15)
  line L220 (123.6813, -64.15) -> (135.5875, -64.15)
  line L221 (230.8375, -64.15) -> (230.8375, -50.15)
  line L222 (170.1813, -49.15) -> (163.1813, -49.15)
  line L223 (95.1062, -50.15) -> (81.1062, -50.15)
  line L224 (211.7875, -64.15) -> (216.8375, -64.15)
  line L225 (178.7375, -50.15) -> (178.7375, -64.15)
  line L226 (192.7375, -64.15) -> (192.7375, -50.15)
  line L227 (197.7875, -50.15) -> (197.7875, -64.15)
  line L228 (170.1813, -64.15) -> (170.1813, -49.15)
  line L229 (209.6937, -50.15) -> (197.7875, -50.15)
  line L230 (211.7875, -50.15) -> (209.6938, -50.15)
  line L231 (216.8375, -50.15) -> (211.7875, -50.15)
  line L232 (209.6937, -64.15) -> (211.7875, -64.15)
  line L233 (103.5442, -49.15) -> (96.5443, -49.15)
  line L234 (96.5443, -64.15) -> (103.5443, -64.15)
  line L235 (95.1062, -64.15) -> (95.1062, -50.15)
  line L236 (152.5437, -50.15) -> (152.5437, -64.15)
  line L237 (154.925, -50.15) -> (152.5438, -50.15)
  line L238 (230.8375, -50.15) -> (223.6938, -50.15)
  line L239 (223.6938, -50.15) -> (216.8375, -50.15)
  line L240 (135.5875, -50.15) -> (123.6813, -50.15)